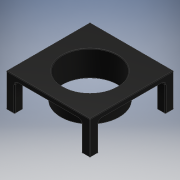
# Autodesk Inventor part: P-POD_Plunger
Saved by Autodesk Inventor 2018 (Build 220112000, 112)
## iProperties
Created: 2018-07-16
Part Number: P-POD_Plunger
Material: Aluminum 6061
Document SubType Name: Modeling
Designer: Bradley
Density: 2.7 g/cm^3
Appearance: Anodized - Dark Gray
Author: Bradley
Autodesk Inventor part; units mm, degrees
ref_plane "YZ Plane" through (0, 0, 0) normal (1, 0, 0) x (0, 1, 0)
ref_plane "XZ Plane" through (0, 0, 0) normal (0, 1, 0) x (-1, 0, 0)
ref_plane "XY Plane" through (0, 0, 0) normal (0, 0, 1) x (1, 0, 0)
sketch "Sketch1" plane through (0, 0, 0) normal (0, 0, 1) x (1, 0, 0)
  line L0 (-50, -50) -> (50, -50)
  line L1 (50, -50) -> (50, 50)
  line L2 (50, 50) -> (-50, 50)
  line L3 (-50, 50) -> (-50, -50)
  line L4 (-50, -50) -> (50, 50) construction
  line L5 (50, -50) -> (-50, 50) construction
  circle A0 centre (0, 0) radius 32.5
  dimension "d0" = 100
  dimension "d1" = 65
  constraints: 12 end point, 2 midpoint, 2 parallel, 2 perpendicular, 1 centre point, 1 coincident, 1 horizontal
  measures "d0" distance of L2.end L1.end
  measures "d1" diameter of A0
extrude "Extrusion1" add sketch "Sketch1" along normal mid plane 40
sketch "Sketch2" plane through (0, 0, -20) normal (0, 0, -1) x (-1, 0, 0)
  circle A0 centre (0, 0) radius 32.5 projected
  line L0 (-50, -50) -> (50, -50) projected
  line L1 (50, -50) -> (50, 50) projected
  line L2 (50, 50) -> (-50, 50) projected
  line L3 (-50, 50) -> (-50, -50) projected
  line L4 (-50, -50) -> (-50, 50) projected
  line L5 (-50, 50) -> (-40, 50)
  line L6 (-40, 50) -> (-40, 40)
  line L7 (-40, 40) -> (-50, 40)
  line L8 (-50, 40) -> (-50, 50)
  line L9 (50, 50) -> (40, 50)
  line L10 (40, 50) -> (40, 40)
  line L11 (40, 40) -> (50, 40)
  line L12 (50, 40) -> (50, 50)
  line L13 (50, -50) -> (-50, -50) projected
  line L14 (50, -50) -> (40, -50)
  line L15 (40, -50) -> (40, -40)
  line L16 (40, -40) -> (50, -40)
  line L17 (50, -40) -> (50, -50)
  line L18 (-50, -50) -> (-40, -50)
  line L19 (-40, -50) -> (-40, -40)
  line L20 (-40, -40) -> (-50, -40)
  line L21 (-50, -40) -> (-50, -50)
  dimension "d4" = 10
  constraints: 32 end point, 8 parallel, 7 perpendicular, 4 collinear, 4 horizontal
  measures "d4" distance of L6.end L7.end
extrude "Extrusion2" cut sketch "Sketch2" against normal blind 34 contours L19 L20 L3 L7 L6 L2 L10 L11 L1 L16 L15 L0
sketch "Sketch3" plane through (0, 0, 14) normal (0, 0, -1) x (-1, 0, 0)
  circle A0 centre (0, 0) radius 32.5 projected
  line L0 (-40, -40) -> (-50, -40) projected
  line L1 (-40, -50) -> (-40, -40) projected
  line L2 (40, -50) -> (-40, -50) projected
  line L3 (40, -40) -> (40, -50) projected
  line L4 (50, -40) -> (40, -40) projected
  line L5 (50, 40) -> (50, -40) projected
  line L6 (40, 40) -> (50, 40) projected
  line L7 (40, 50) -> (40, 40) projected
  line L8 (-40, 50) -> (40, 50) projected
  line L9 (-40, 40) -> (-40, 50) projected
  line L10 (-50, 40) -> (-40, 40) projected
  line L11 (-50, -40) -> (-50, 40) projected
  circle A1 centre (0, 0) radius 35
  dimension "d7" = 70
  constraints: 1 centre point, 1 coincident
  measures "d7" diameter of A1
extrude "Extrusion3" add sketch "Sketch3" along normal blind 25 contours A1
fillet "Fillet1" radius 4 9 edges at (45, 40, 14) (40, 45, 14) (-40, 45, 14) (-45, 40, 14) (-40, -45, 14) (-45, -40, 14) (40, -45, 14) (45, -40, 14) (35, 0, 14)
fillet "Fillet1" radius 0.7 43 edges at (0, -50, 20) (50, 0, 20) (0, 50, 20) (-50, 0, 20) (50, -40, -3) (50, 0, 14) (50, 40, -3) (50, 45, -20) (50, 50, 0) (50, -50, 0) (50, -45, -20) (40, 50, -3) (0, 50, 14) (-40, 50, -3) (-45, 50, -20) (-50, 50, 0) (45, 50, -20) (-50, -40, -3) (-50, -45, -20) (-50, -50, 0) (-50, 45, -20) (-50, 40, -3) (-50, 0, 14) (-40, -50, -3) (0, -50, 14) (40, -50, -3) (45, -50, -20) (-45, -50, -20) (-40, -45, -20) (-40, -40, -3) (-45, -40, -20) (-40, 45, -20) (-40, 40, -3) (-45, 40, -20) (40, 45, -20) (40, 40, -3) (45, 40, -20) (45, -40, -20) (40, -40, -3) (40, -45, -20) (35, 0, -11) (32.5, 0, -11) (-32.5, 0, 20)
body "Solid1"
